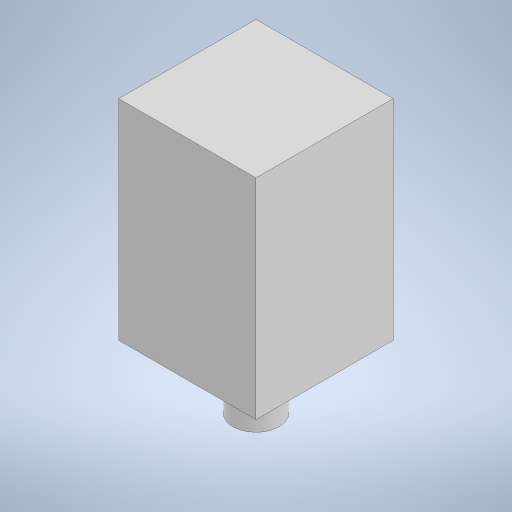
# Autodesk Inventor part: Motor
Saved by Autodesk Inventor 2024 (Build 280153000, 153)
## iProperties
Created: 2024-10-17
Part Number: Motor
Material: Genérico
Document SubType Name: Modeling
Designer: robof
Density: 1 g/cm^3
Appearance: Padrão
Author: robof
Autodesk Inventor part; units mm, degrees
ref_plane "YZ Plane" through (0, 0, 0) normal (1, 0, 0) x (0, 1, 0)
ref_plane "XZ Plane" through (0, 0, 0) normal (0, 1, 0) x (-1, 0, 0)
ref_plane "XY Plane" through (0, 0, 0) normal (0, 0, 1) x (1, 0, 0)
sketch "Esboço1" plane through (0, 0, 0) normal (0, 1, 0) x (-1, 0, 0)
  circle A0 centre (0, 0) radius 9.5
  dimension "d2" = 19
  constraints: 1 centre point, 1 coincident
  measures "d2" diameter of A0
extrude "Extrusão1" add sketch "Esboço1" along normal blind 26
sketch "Esboço2" plane through (0, 26, 0) normal (0, 1, 0) x (1, 0, 0)
  line L0 (0, 0) -> (-28.2, 0)
  line L1 (-28.2, 0) -> (-28.2, 28.2)
  line L2 (-28.2, 28.2) -> (0, 28.2)
  line L3 (0, 28.2) -> (0, 0)
  line L4 (-28.2, 28.2) -> (28.2, 28.2)
  line L5 (28.2, 28.2) -> (28.2, -28.2)
  line L6 (28.2, -28.2) -> (-28.2, -28.2)
  line L7 (-28.2, -28.2) -> (-28.2, 28.2)
  dimension "d5" = 28.2
  dimension "d6" = 28.2
  dimension "d7" = 56.4
  dimension "d8" = 56.4
  constraints: 16 end point, 4 parallel, 2 horizontal, 2 perpendicular
  measures "d5" distance of L1.end L2.end
  measures "d6" distance of L0.end L1.end
  measures "d7" distance of L5.end L6.end
  measures "d8" distance of L4.end L5.end
extrude "Extrusão2" add sketch "Esboço2" along normal blind 86
